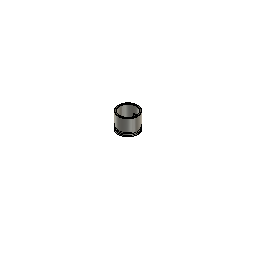
Festool_Dust_Adapter_CNC_2_v4 (Autodesk Fusion 360 design; units mm, degrees)
Autodesk Fusion 360 part; units mm, degrees
sketch "Sketch1" plane through (0, 0, 0) normal (0, 0, 1) x (1, 0, 0)
  circle A0 centre (0, 0) radius 18.25
  circle A1 centre (0, 0) radius 22
  dimension "d67" = 36.5
  dimension "d68" = 44
  measures "d67" diameter of A0
  measures "d68" diameter of A1
extrude "Extrude1" add sketch "Sketch1" along normal blind 36
sketch "Sketch2" plane through (0, 0, 0) normal (1, 0, 0) x (0, 1, 0)
  line L0 (18.25, 19) -> (17.15, 19)
  line L1 (17.15, 19) -> (17.15, 12)
  line L2 (17.15, 12) -> (18.25, 12)
  line L3 (18.25, 12) -> (18.25, 19)
  line L4 (-18.25, 36) -> (18.25, 36)
  line L5 (-18.25, 0) -> (18.25, 0)
  dimension "d71" = 17
  dimension "d72" = 1.1
  dimension "d73" = 7
revolve "Revolve1" add sketch "Sketch2" angle 15 about axis through (0, 0, -205.75) along (0, 0, -1) second angle 15
pattern_circular "C-Pattern1" count 3 over 360 about axis through (0, 0, -205.75) along (0, 0, 1) of "Revolve1"
sketch "Sketch3" plane through (0, 0, 0) normal (0, 0, -1) x (1, 0, 0)
  circle A0 centre (0, 0) radius 18.25
  circle A1 centre (0, 0) radius 22
  circle A2 centre (0, 0) radius 20
  dimension "d78" = 40
  measures "d78" diameter of A2
extrude "Extrude2" cut sketch "Sketch3" against normal blind 8 contours A2
thread "Thread1" "ISO Metric profile 42.0 M42x3 6H" major diameter 42.349 minor diameter 39.0024 pitch 3 angle 60 modelled right hand crest width 0.375 on face at (19.9751, 0.9969, 5.3333) crest through (19.5012, 0, -1.6875)
chamfer "Chamfer1" distance 0.6 angle 45 2 edges at (-20.5112, -7.9555, 36) (-17.015, 6.5995, 36)
fillet "Fillet1" radius 0.8 24 edges at (14.8523, -8.575, 19) (16.5656, -4.4387, 15.5) (12.1269, -12.1269, 15.5) (12.5158, -12.5158, 19) (17.0969, -4.5811, 19) (14.8523, -8.575, 12) (12.5158, -12.5158, 12) (17.0969, -4.5811, 12) (-14.8523, -8.575, 19) (-12.1269, -12.1269, 15.5) (-14.8523, -8.575, 12) (-16.5656, -4.4387, 15.5) (-17.0969, -4.5811, 19) (-12.5158, -12.5158, 19) (-12.5158, -12.5158, 12) (-17.0969, -4.5811, 12) (0, 17.15, 19) (4.4387, 16.5656, 15.5) (4.5811, 17.0969, 19) (-4.5811, 17.0969, 19) (-4.4387, 16.5656, 15.5) (0, 17.15, 12) (4.5811, 17.0969, 12) (-4.5811, 17.0969, 12)
equation "d67 = ( 18.25 * 2 ) * 1 mm"
